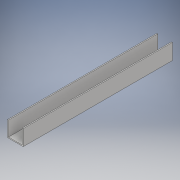
# Autodesk Inventor part: BeamSolid1
Saved by Autodesk Inventor 2017 (Build 210142000, 142)
## iProperties
Created: 2016-09-18
Part Number: BeamSolid1
Material: Generic
Document SubType Name: Modeling
Designer: Spartacles
Density: 1 g/cm^3
Appearance: Default
Author: Spartacles
Autodesk Inventor part; units mm, degrees
ref_plane "YZ Plane" through (0, 0, 0) normal (1, 0, 0) x (0, 1, 0)
ref_plane "XZ Plane" through (0, 0, 0) normal (0, 1, 0) x (-1, 0, 0)
ref_plane "XY Plane" through (0, 0, 0) normal (0, 0, 1) x (1, 0, 0)
sketch "Sketch1" plane through (0, 0, 0) normal (0, 0, 1) x (1, 0, 0)
  line L0 (2.0066, 32.004) -> (0, 32.004)
  line L1 (0, 32.004) -> (0, 0)
  line L2 (0, 0) -> (2.0066, 0)
  line L3 (2.0066, 2.0066) -> (2.0066, 32.004)
  line L4 (2.0066, 0) -> (29.9974, 0)
  line L5 (29.9974, 2.0066) -> (2.0066, 2.0066)
  line L6 (29.9974, 0) -> (32.004, 0)
  line L7 (32.004, 0) -> (32.004, 32.004)
  line L8 (32.004, 32.004) -> (29.9974, 32.004)
  line L9 (29.9974, 32.004) -> (29.9974, 2.0066)
  dimension "d2" = 2.0066
  dimension "d3" = 32.004
  constraints: 20 end point, 5 parallel, 3 horizontal, 2 perpendicular
  measures "d2" distance of L8.end L7.end
  measures "d3" distance of L7.end L6.end
sketch "Sketch2" plane through (0, 0, 0) normal (0, 0, 1) x (1, 0, 0)
  point P0 (0, 0)
extrude "Extrusion1" add sketch "Sketch1" along normal blind 304.8
body "Solid1"
